Autodesk Inventor part; units mm, degrees
(part 3 of 3)
sketch "スケッチ20" plane through (0, 0, -2) normal (0, 0, 1) x (1, 0, 0)
  arc A0 (80.70524, -27.111077) -> (82.046941, -27.063125) centre (81.349617, -26.346369) ccw
  line L0 (82.046941, -27.063125) -> (98.043988, -11.499772)
  arc A1 (98.043988, -11.499772) -> (97.055271, -9.826413) centre (97.346664, -10.783016) ccw
  arc A2 (93.489695, -9.2) -> (97.055271, -9.826413) centre (95.889695, -6) ccw
  arc A3 (93.489695, -9.2) -> (92.889695, -9) centre (92.889695, -10) ccw
  line L1 (92.889695, -9) -> (91.889695, -9)
  arc A4 (91.889695, -9) -> (91.289695, -9.2) centre (91.889695, -10) ccw
  arc A5 (85.217782, -7.586522) -> (91.289695, -9.2) centre (88.889695, -6) ccw
  arc A6 (85.217782, -7.586522) -> (84.217782, -6.986522) centre (84.299804, -7.983153) ccw
  arc A7 (81.489695, -6.2) -> (84.217782, -6.986522) centre (83.889695, -3) ccw
  arc A8 (81.489695, -6.2) -> (80.889695, -6) centre (80.889695, -7) ccw
  line L2 (80.889695, -6) -> (73.444342, -6)
  arc A9 (73.444342, -6) -> (72.844342, -6.2) centre (73.444342, -7) ccw
  arc A10 (70.116255, -6.986522) -> (72.844342, -6.2) centre (70.444342, -3) ccw
  arc A11 (70.116255, -6.986522) -> (69.116255, -7.586522) centre (70.034233, -7.983153) ccw
  arc A12 (63.044342, -9.2) -> (69.116255, -7.586522) centre (65.444342, -6) ccw
  arc A13 (63.044342, -9.2) -> (62.444342, -9) centre (62.444342, -10) ccw
  line L3 (62.444342, -9) -> (61.950732, -9)
  arc A14 (61.950732, -9) -> (61.306355, -10.764708) centre (61.950732, -10) ccw
  line L4 (61.306355, -10.764708) -> (80.70524, -27.111077)
  arc A15 (100.885049, -15.289324) -> (99.187725, -14.572568) centre (99.885049, -15.289324) ccw
  line L5 (99.187725, -14.572568) -> (84.49462, -28.86733)
  arc A16 (84.49462, -28.86733) -> (84.547567, -30.348794) centre (85.191944, -29.584086) ccw
  line L6 (84.547567, -30.348794) -> (97.304324, -41.098208)
  arc A17 (97.304324, -41.098208) -> (98.944155, -40.238251) centre (97.948701, -40.3335) ccw
  arc A18 (100.742192, -32.303978) -> (98.944155, -40.238251) centre (111.885049, -39.000002) ccw
  arc A19 (100.742192, -32.303978) -> (100.885049, -31.788899) centre (99.885049, -31.788899) ccw
  line L7 (100.885049, -31.788899) -> (100.885049, -15.289324)
  arc A20 (61.161301, -51.568062) -> (61.858625, -53.284818) centre (61.858625, -52.284818) ccw
  line L8 (61.858625, -53.284818) -> (102.968005, -53.284818)
  arc A21 (102.968005, -53.284818) -> (103.525321, -51.454517) centre (102.968005, -52.284818) ccw
  arc A22 (102.219392, -50.47062) -> (103.525321, -51.454517) centre (111.885049, -39.000002) ccw
  line L9 (102.219392, -50.47062) -> (81.514654, -33.023881)
  arc A23 (81.514654, -33.023881) -> (80.172953, -33.071833) centre (80.870277, -33.788589) ccw
  line L10 (80.172953, -33.071833) -> (61.161301, -51.568062)
  circle A24 centre (90.019865, -69.833545) radius 1.5
  circle A25 centre (49.97225, -10.5) radius 1.5
  line L11 (58.301358, -15.613652) -> (58.301358, -47.79688)
  arc A26 (58.301358, -47.79688) -> (59.998682, -48.513636) centre (59.301358, -47.79688) ccw
  line L12 (59.998682, -48.513636) -> (77.725274, -31.267628)
  arc A27 (77.725274, -31.267628) -> (77.672327, -29.786164) centre (77.02795, -30.550872) ccw
  line L13 (77.672327, -29.786164) -> (59.945735, -14.848944)
  arc A28 (59.945735, -14.848944) -> (58.301358, -15.613652) centre (59.301358, -15.613652) ccw
  arc A29 (63.926064, -84.906051) -> (65.171844, -84.473428) centre (64.30232, -83.979536) ccw
  arc A30 (72.586796, -76.717312) -> (65.171844, -84.473428) centre (84.301358, -95.339048) ccw
  line L14 (72.586796, -76.717312) -> (85.450729, -68.62487)
  arc A31 (85.450729, -68.62487) -> (85.845815, -68.152085) centre (84.918248, -67.778427) ccw
  arc A32 (90.311221, -65.342987) -> (85.845815, -68.152085) centre (90.019865, -69.833545) ccw
  arc A33 (90.311221, -65.342987) -> (90.908447, -65.191528) centre (90.375967, -64.345086) ccw
  line L15 (90.908447, -65.191528) -> (102.131611, -58.13126)
  arc A34 (102.131611, -58.13126) -> (101.599131, -56.284818) centre (101.599131, -57.284818) ccw
  line L16 (101.599131, -56.284818) -> (59.301358, -56.284818)
  arc A35 (59.301358, -56.284818) -> (58.301358, -57.284818) centre (59.301358, -57.284818) ccw
  line L17 (58.301358, -57.284818) -> (58.301358, -81.948654)
  arc A36 (58.301358, -81.948654) -> (58.925101, -82.875169) centre (59.301358, -81.948654) ccw
  line L18 (58.925101, -82.875169) -> (63.926064, -84.906051)
  arc A37 (63.012459, -89.790822) -> (62.743712, -90.949526) centre (84.301358, -95.339048) ccw
  arc A38 (63.012459, -89.790822) -> (62.421039, -88.612114) centre (62.044782, -89.538629) ccw
  line L19 (62.421039, -88.612114) -> (57.363161, -86.558119)
  arc A39 (57.363161, -86.558119) -> (56.372647, -86.695529) centre (56.986905, -87.484634) ccw
  arc A40 (54.195568, -87.669391) -> (56.372647, -86.695529) centre (53.301358, -82.750002) ccw
  arc A41 (54.195568, -87.669391) -> (53.376337, -88.591228) centre (54.374411, -88.653269) ccw
  arc A42 (53.120069, -89.942419) -> (53.376337, -88.591228) centre (47.886932, -88.250002) ccw
  arc A43 (53.120069, -89.942419) -> (53.691557, -91.175122) centre (54.071549, -90.250132) ccw
  line L20 (53.691557, -91.175122) -> (54.908362, -91.674992)
  arc A44 (54.908362, -91.674992) -> (55.288353, -91.750002) centre (55.288353, -90.750002) ccw
  line L21 (55.288353, -91.750002) -> (61.763819, -91.750002)
  arc A45 (61.763819, -91.750002) -> (62.743712, -90.949526) centre (61.763819, -90.750002) ccw
  circle A46 centre (47.886932, -88.250002) radius 1.5
  line L22 (104.885049, -3) -> (104.885049, -31.858573)
  arc A47 (104.885049, -31.858573) -> (119.12697, -45.895985) centre (111.885049, -39.000002) ccw
  line L23 (119.12697, -45.895985) -> (127.651316, -45.772687)
  line L24 (127.651316, -45.772687) -> (121.057661, -50.868582)
  arc A48 (119.87225, -51.69664) -> (121.057661, -50.868582) centre (111.885049, -39.000002) ccw
  line L25 (119.87225, -51.69664) -> (94.777748, -67.483089)
  arc A49 (94.777748, -67.483089) -> (94.348344, -68.602989) centre (95.310228, -68.329531) ccw
  arc A50 (87.036679, -73.202611) -> (94.348344, -68.602989) centre (90.019865, -69.833545) ccw
  arc A51 (87.036679, -73.202611) -> (85.841268, -73.104849) centre (86.373748, -73.951292) ccw
  line L26 (85.841268, -73.104849) -> (74.716716, -80.103082)
  arc A52 (74.716716, -80.103082) -> (66.301358, -95.339048) centre (84.301358, -95.339048) ccw
  line L27 (66.301358, -95.339048) -> (66.301358, -95.750002)
  line L28 (66.301358, -95.750002) -> (54.301358, -95.750002)
  line L29 (54.301358, -95.750002) -> (46.176972, -92.412457)
  arc A53 (47.886932, -83.750002) -> (46.176972, -92.412457) centre (47.886932, -88.250002) ccw
  line L30 (47.886932, -83.750002) -> (53.301358, -83.750002)
  arc A54 (53.301358, -83.750002) -> (54.301358, -82.750002) centre (53.301358, -82.750002) ccw
  line L31 (54.301358, -82.750002) -> (54.301358, -14.878018)
  arc A55 (54.301358, -14.878018) -> (52.696065, -14.082015) centre (53.301358, -14.878018) ccw
  arc A56 (48.722143, -6.177127) -> (52.696065, -14.082015) centre (49.97225, -10.5) ccw
  arc A57 (48.722143, -6.177127) -> (49.444342, -5.216488) centre (48.444342, -5.216488) ccw
  line L32 (49.444342, -6.031072) -> (49.444342, -5.216488)
  arc A58 (52.715827, -6.933099) -> (49.444342, -6.031072) centre (49.97225, -10.5) ccw
  arc A59 (52.715827, -6.933099) -> (53.329954, -6.998364) centre (53.444342, -3) ccw
  arc A60 (54.301358, -7.997955) -> (53.329954, -6.998364) centre (53.301358, -7.997955) ccw
  line L33 (54.301358, -14.878018) -> (54.301358, -7.997955)
  line L34 (101.889695, -3) -> (104.885049, -3)
  arc A61 (99.889695, -3) -> (101.889695, -3) centre (100.889695, -3) ccw
  line L35 (99.889695, 0) -> (99.889695, -3)
  line L36 (84.889695, 0) -> (99.889695, 0)
  line L37 (84.889695, -3) -> (84.889695, 0)
  arc A62 (82.889695, -3) -> (84.889695, -3) centre (83.889695, -3) ccw
  line L38 (71.444342, -3) -> (82.889695, -3)
  arc A63 (69.444342, -3) -> (71.444342, -3) centre (70.444342, -3) ccw
  line L39 (66.444342, -3) -> (69.444342, -3)
  line L40 (66.444342, -6) -> (66.444342, -3)
  arc A64 (64.444342, -6) -> (66.444342, -6) centre (65.444342, -6) ccw
  line L41 (59.444342, -6) -> (64.444342, -6)
  arc A65 (57.444342, -6) -> (59.444342, -6) centre (58.444342, -6) ccw
  line L42 (57.444342, -3) -> (57.444342, -6)
  line L43 (54.444342, -3) -> (57.444342, -3)
  line L44 (54.444342, -3) -> (54.444342, 0)
  line L45 (54.444342, 0) -> (69.444342, 0)
  line L46 (69.444342, 0) -> (69.444342, -3)
  line L47 (49.444342, -5.216488) -> (49.444342, -3)
  line L48 (49.444342, -3) -> (52.444342, -3)
  arc A66 (52.444342, -3) -> (54.444342, -3) centre (53.444342, -3) ccw
  line L49 (96.889695, -3) -> (99.889695, -3)
  line L50 (96.889695, -6) -> (96.889695, -3)
  arc A67 (94.889695, -6) -> (96.889695, -6) centre (95.889695, -6) ccw
  line L51 (89.889695, -6) -> (94.889695, -6)
  arc A68 (87.889695, -6) -> (89.889695, -6) centre (88.889695, -6) ccw
  line L52 (87.889695, -3) -> (87.889695, -6)
  arc A69 (89.889695, -3) -> (87.889695, -3) centre (88.889695, -3) ccw
  line L53 (94.889695, -3) -> (89.889695, -3)
  arc A70 (96.889695, -3) -> (94.889695, -3) centre (95.889695, -3) ccw
  line L54 (84.889695, -3) -> (87.889695, -3)
  arc A71 (66.444342, -3) -> (64.444342, -3) centre (65.444342, -3) ccw
  line L55 (64.444342, -3) -> (59.444342, -3)
  arc A72 (59.444342, -3) -> (57.444342, -3) centre (58.444342, -3) ccw
  circle A73 centre (49.97225, -10.5) radius 1.5
  circle A74 centre (49.97225, -10.5) radius 3
  point P0 (0, 0)
  dimension "d177" = 6
  constraints: 1 centre point, 1 coincident
  measures "d177" diameter of A74
extrude "押し出し26" cut sketch "スケッチ20" against normal blind 0.4 contours A74
equation "\"d9\" = d7"
equation "\"d26\" = d7"
